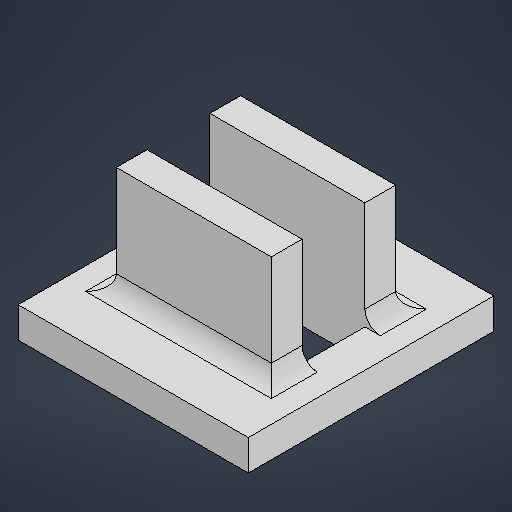
# Autodesk Inventor part: LRA_case1
Saved by Autodesk Inventor 2026 (Build 300175050, 175E)
## iProperties
Created: 2025-09-05
Part Number: LRA_case1
Material: 一般
Document SubType Name: Modeling
Designer: ka0n7
Density: 1 g/cm^3
Appearance: 既定
Author: ka0n7
Autodesk Inventor part; units mm, degrees
ref_plane "YZ Plane" through (0, 0, 0) normal (1, 0, 0) x (0, 1, 0)
ref_plane "XZ Plane" through (0, 0, 0) normal (0, 1, 0) x (-1, 0, 0)
ref_plane "XY Plane" through (0, 0, 0) normal (0, 0, 1) x (1, 0, 0)
sketch "スケッチ1" plane through (0, 0, 0) normal (0, 1, 0) x (-1, 0, 0)
  line L0 (7.5, 8) -> (-7.5, 8)
  line L1 (-7.5, 8) -> (-7.5, -8)
  line L2 (-7.5, -8) -> (7.5, -8)
  line L3 (7.5, -8) -> (7.5, 8)
  line L4 (7.5, 8) -> (-7.5, -8) construction
  line L5 (-7.5, 8) -> (7.5, -8) construction
  line L6 (5.05, 2.05) -> (-5.05, 2.05)
  line L7 (-5.05, 2.05) -> (-5.05, -2.05)
  line L8 (-5.05, -2.05) -> (5.05, -2.05)
  line L9 (5.05, -2.05) -> (5.05, 2.05)
  line L10 (5.05, 2.05) -> (-5.05, -2.05) construction
  line L11 (-5.05, 2.05) -> (5.05, -2.05) construction
  point P0 (0, 0)
  dimension "d0" = 15
  dimension "d1" = 16
  dimension "d2" = 10.1
  dimension "d3" = 4.1
  constraints: 24 end point, 4 midpoint, 4 parallel, 2 horizontal, 2 perpendicular
  measures "d0" distance of L2.end L1.end
  measures "d1" distance of L2.end L0.start
  measures "d2" distance of L8.end L7.end
  measures "d3" distance of L6.end L7.end
extrude "押し出し1" add sketch "スケッチ1" along normal blind 2
sketch "スケッチ2" plane through (0, 2, 0) normal (0, 1, 0) x (1, 0, 0)
  line L0 (-5.05, 2.05) -> (5.05, 2.05) projected
  line L1 (-5.05, 2.05) -> (5.05, 2.05)
  line L2 (5.05, 2.05) -> (5.05, 4.05)
  line L3 (5.05, 4.05) -> (-5.05, 4.05)
  line L4 (-5.05, 4.05) -> (-5.05, 2.05)
  line L5 (5.05, -2.05) -> (-5.05, -2.05) projected
  line L6 (-5.05, -2.05) -> (5.05, -2.05)
  line L7 (5.05, -2.05) -> (5.05, -4.05)
  line L8 (5.05, -4.05) -> (-5.05, -4.05)
  line L9 (-5.05, -4.05) -> (-5.05, -2.05)
  point P0 (0, 0)
  point P1 (5.05, 2.05)
  dimension "d6" = 2
  dimension "d7" = 2
  constraints: 16 end point, 4 parallel, 2 horizontal, 2 perpendicular, 1 point on line
  measures "d6" distance of L3.end L0.start
  measures "d7" distance of L8.end L5.end
extrude "押し出し2" add sketch "スケッチ2" along normal blind 7
fillet "フィレット1" radius 1 6 edges at (5.05, 2, 3.05) (0, 2, 4.05) (-5.05, 2, 3.05) (-5.05, 2, -3.05) (0, 2, -4.05) (5.05, 2, -3.05)
equation "\"d7\" = d6"
